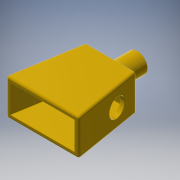
# Autodesk Inventor part: Cuerpo Lego
Saved by Autodesk Inventor 2017 (Build 210142000, 142)
## iProperties
Created: 2017-06-23
Part Number: Cuerpo Lego
Material: Plástico ABS
Document SubType Name: Modeling
Designer: H. Valenzuela B.
Density: 1.06 g/cm^3
Appearance: Suave - Blanco
Author: H. Valenzuela B.
Autodesk Inventor part; units mm, degrees
ref_plane "YZ Plane" through (0, 0, 0) normal (1, 0, 0) x (0, 1, 0)
ref_plane "XZ Plane" through (0, 0, 0) normal (0, 1, 0) x (-1, 0, 0)
ref_plane "XY Plane" through (0, 0, 0) normal (0, 0, 1) x (1, 0, 0)
sketch "Boceto1" plane through (0, 0, 0) normal (0, 0, 1) x (1, 0, 0)
  line L0 (0, 18.2) -> (0, -4.2) construction
  line L1 (-11.2, 0) -> (11.2, 0) construction
  line L2 (-8, 0) -> (-5.5, 15)
  line L3 (-5.5, 15) -> (5.5, 15)
  line L4 (5.5, 15) -> (8, 0)
  line L5 (-8, 0) -> (8, 0)
  line L6 (-8, 0) -> (8, 0)
  line L7 (8, 0) -> (8, -1) construction
  line L8 (8, -1) -> (-8, -1) construction
  line L9 (-8, -1) -> (-8, 0) construction
  point P0 (0, 0)
  point P1 (-5.5, 15)
  point P2 (5.5, 15)
  dimension "d3" = 0
  dimension "d0" = 11
  dimension "d1" = 15
  dimension "d2" = 16
  dimension "d4" = 1
  constraints: 16 end point, 7 point on line, 4 horizontal, 3 parallel, 1 perpendicular, 11 other
  measures "d0" distance of point (-5.5, 15) point (5.5, 15)
  measures "d1" distance between parallel lines of L1 L3
  measures "d2" distance of L2.start L4.end
  measures "d4" distance of L6.end L7.end
extrude "Extrusión1" add sketch "Boceto1" along normal mid plane 8
shell "Vaciado1" thickness 1 removed faces 1 at (2.6667, 0, 1.3333)
sketch "Boceto2" plane through (0, 0, 0) normal (1, 0, 0) x (0, 1, 0)
  line L0 (-4.16, 0) -> (24.96, 0) projected
  line L1 (15, 2.225) -> (20.8, 2.225)
  line L2 (20.8, 2.225) -> (20.8, 1.5)
  line L3 (20.8, 1.5) -> (15, 1.5)
  line L4 (15, 1.5) -> (15, 2.225)
  line L5 (15, -4) -> (15, 4) projected
  point P0 (0, 0)
  dimension "d8" = 5.8
  dimension "d9" = 4.45
  dimension "d10" = 3
  constraints: 8 end point, 2 parallel, 1 collinear, 1 horizontal, 1 perpendicular
  measures "d8" distance of L1.start L1.end
  measures "d9" diameter of L1 L0
  measures "d10" diameter of L3 L0
revolve "Revolución1" add sketch "Boceto2" angle 360 about axis through (0, -10, 0) along (0, 1, 0)
sketch "Boceto3" plane through (0, 0, 0) normal (1, 0, 0) x (0, 1, 0)
  line L0 (-3, 0) -> (18, 0) construction
  circle A0 centre (10, 0) radius 2
  line L1 (15, -4) -> (15, 4) projected
  point P0 (0, 0)
  dimension "d12" = 4
  dimension "d17" = 5
  constraints: 1 centre point, 1 point on line
  measures "d12" diameter of A0
  measures "d17" distance from line of L1 A0.centre
extrude "Extrusión2" cut sketch "Boceto3" along normal through all both and the other way through all
fillet "Empalme1" radius 0.5 12 edges at (-6.75, 7.5, -4) (0, 15, -4) (6.75, 7.5, -4) (-8, 0, 0) (-6.75, 7.5, 4) (6.75, 7.5, 4) (8, 0, 0) (0, 15, 4) (0, 0, 4) (0, 0, -4) (-5.5, 15, 0) (5.5, 15, 0)
fillet "Empalme2" radius 0.1 10 edges at (5.8195, 7, -3) (0, 14, -3) (-5.8195, 7, -3) (-4.6529, 14, 0) (-5.8195, 7, 3) (4.6529, 14, 0) (0, 14, 3) (5.8195, 7, 3) (0, 20.8, -1.5) (0, 20.8, -2.225)
fillet "Empalme3" radius 0.1 4 edges at (6.6667, 8, 0) (5.6529, 8, 0) (-6.6667, 8, 0) (-5.6529, 8, 0)
fillet "Empalme4" radius 0.1 1 edges at (0, 15, -2.225)
fillet "Empalme5" radius 0.1 8 edges at (-6.9565, 0, -2.9707) (-6.9862, 0, 0) (-6.9565, 0, 2.9707) (0, 0, 3) (6.9565, 0, 2.9707) (6.9862, 0, 0) (6.9565, 0, -2.9707) (0, 0, -3)
